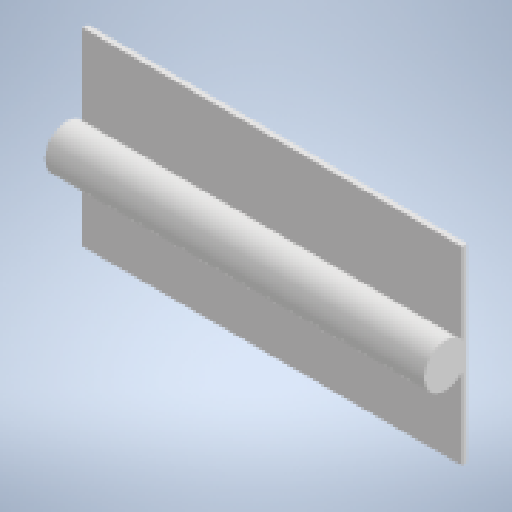
# Autodesk Inventor part: charnière
Saved by Autodesk Inventor 2024.2 (Build 282272000, 272)
## iProperties
Created: 2024-10-04
Part Number: charnière
Material: Générique
Document SubType Name: Modeling
Designer: Sebastien
Density: 1 g/cm^3
Appearance: Par défaut
Author: Sebastien
Autodesk Inventor part; units mm, degrees
ref_plane "YZ Plane" through (0, 0, 0) normal (1, 0, 0) x (0, 1, 0)
ref_plane "XZ Plane" through (0, 0, 0) normal (0, 1, 0) x (-1, 0, 0)
ref_plane "XY Plane" through (0, 0, 0) normal (0, 0, 1) x (1, 0, 0)
sketch "Esquisse1" plane through (0, 0, 0) normal (1, 0, 0) x (0, 1, 0)
  line L0 (24, 0) -> (24, 1)
  line L1 (24, 1) -> (2.6458, 1)
  line L2 (24, 0) -> (0, 0)
  line L3 (0, 0) -> (0, 8)
  arc A0 (0, 0) -> (2.6458, 1) centre (0, 4) ccw construction
  arc A1 (2.6458, 1) -> (0, 8) centre (0, 4) ccw
  dimension "d0" = 1
  dimension "d1" = 48
  dimension "d2" = 4
  constraints: 8 end point, 4 point on circle, 2 centre point, 2 vertical, 1 coincident, 1 horizontal, 1 midpoint, 1 perpendicular
  measures "d0" distance of L0.start L0.end
  measures "d1" diameter of L0 L3
  measures "d2" radius of A1
extrude "Extrusion1" add sketch "Esquisse1" along normal mid plane 100
mirror "Mise en miroir1" about plane through (0, 0, 0) normal (0, 1, 0)
